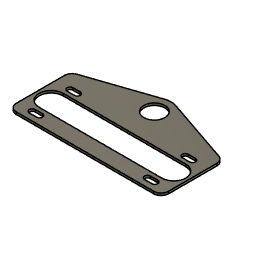
IntakeBack v1 (Autodesk Fusion 360 design; units mm, degrees)
Autodesk Fusion 360 part; units mm, degrees
note: some values were not read from the file. Set by a fixed rule: which sketch regions a step uses.
sketch "Sketch1" plane through (0, 0, 0) normal (0, 1, 0) x (1, 0, 0)
  circle A0 centre (-75, 25) radius 4
  circle A1 centre (-75, -25.8) radius 4
  circle A2 centre (90.1, 25) radius 4
  circle A3 centre (90.1, -25.8) radius 4
  circle A4 centre (-75, -0.4) radius 14.224
  circle A5 centre (90.1, -0.4) radius 14.224
  circle A6 centre (7.55, 56.0402) radius 14.224
  line L0 (-95, -37.4041) -> (-95, 45)
  line L1 (-95, 45) -> (110.1, 45)
  line L2 (110.1, 45) -> (110.1, -45.8)
  circle A7 centre (7.55, 56.0402) radius 22.5
  line L3 (-95, 45) -> (0.3196, 77.3468)
  line L4 (110.1, 45) -> (14.7804, 77.3468)
  line L5 (110.1, -45.8) -> (110.1, -37.4041)
  line L6 (110.1, -37.4041) -> (-95, -37.4041)
  line L7 (90.1, -25.8) -> (86.1, -25.8)
  line L8 (-71, -25.8) -> (-75, -25.8)
  line L9 (-75, 25) -> (-75, 21)
  line L10 (-75, -25.8) -> (-75, -21.8)
  line L11 (-75, 13.824) -> (-75, 25)
  line L12 (-75, 25) -> (-71, 25)
  line L13 (86.1, 25) -> (90.1, 25)
  arc A8 (14.7226, 43.7571) -> (14.1002, 45) centre (-75, -0.4) ccw
  arc A9 (0.9998, 45) -> (0.3774, 43.7571) centre (90.1, -0.4) ccw
  line L14 (90.1, 25) -> (90.1, 21)
  line L15 (90.1, -21.8) -> (90.1, -25.8)
  dimension "d1" = 8
  dimension "d2" = 50.8
  dimension "d3" = 8
  dimension "d4" = 165.1
  dimension "d5" = 50.8
  dimension "d6" = 8
  dimension "d7" = 8
  dimension "d8" = 28.448
  dimension "d9" = 28.448
  dimension "d10" = 200
  dimension "d12" = 28.448
  dimension "d14" = 45
  constraint coincident A0.centre L9.start
  constraint vertical L9
  constraint horizontal L12
  constraint vertical L14
  constraint horizontal L7
  constraint vertical L10
  constraint coincident A2.centre L13.end
  constraint coincident A3.centre L7.start
  constraint concentric A4 A8
  constraint coincident A6.centre A8
  constraint concentric A6 A7
  constraint coincident A7 L3.end
  constraint tangent A7 L3
  constraint coincident A7 L4.end
  constraint tangent A7 L4
  constraint vertical L5
  constraint horizontal L6
  constraint coincident L2 L5.end
  constraint coincident A3 L7.end
  constraint collinear L7 L8
  constraint coincident A1 L8.start
  constraint coincident A4.centre L9
  constraint coincident A4 L11.start
  constraint collinear L10 L11
  constraint coincident A1 L10.end
  constraint coincident A0 L9.end
  constraint coincident A0 L12.end
  constraint collinear L12 L13
  constraint coincident A2 L13.start
  constraint coincident A6 A9.end
  constraint coincident A6 A8.start
  constraint coincident L1 A8.end
  constraint coincident L1 A9.start
  constraint coincident A2 L14.end
  constraint collinear L14 L15
  constraint coincident A5.centre L14
  constraint coincident A3 L15.start
  measures "d1" diameter of A0
  measures "d2" distance of A0.centre A1.centre
  measures "d3" diameter of A1
  measures "d4" distance of A0.centre A2.centre
  measures "d5" distance of A0.centre A1.centre
  measures "d6" diameter of A2
  measures "d7" diameter of A3
  measures "d8" diameter of A4
  measures "d9" diameter of A5
  measures "d10" diameter of A8
  measures "d12" diameter of A6
  measures "d14" diameter of A7
extrude "Extrude1" add sketch "Sketch1" along normal blind 3 contours A6 L1 A7 | A6 L1 A7 | L0 L1 L2 A7 L6 | L1 A7 L3 | L1 A7 L4
sketch "Sketch2" plane through (0, 3, 0) normal (0, 1, 0) x (-1, 0, 0)
  circle A0 centre (-90.1, -25) radius 4
  circle A1 centre (-90.1, 0.4) radius 14.224
  circle A2 centre (75, -25) radius 4
  circle A3 centre (75, 25.8) radius 4
  circle A4 centre (75, 0.4) radius 14.224
  circle A5 centre (-90.1, 25.8) radius 4
  circle A6 centre (-7.55, -56.0402) radius 14.224
  line L0 (-110.1, -45) -> (-14.7804, -77.3468)
  arc A7 (-14.7804, -77.3468) -> (-0.3196, -77.3468) centre (-7.55, -56.0402) ccw
  line L1 (-0.3196, -77.3468) -> (95, -45)
  line L2 (95, -45) -> (95, 37.4041)
  line L3 (95, 37.4041) -> (-110.1, 37.4041)
  line L4 (-110.1, 37.4041) -> (-110.1, -45)
  line L5 (75.0984, -13.8237) -> (-90.1, -13.824)
  line L6 (-90.1, 14.624) -> (75, 14.624)
  constraint coincident A4 L5.start
  constraint coincident A1 L5.end
  constraint tangent A1 L5
  constraint coincident A1 L6.start
  constraint coincident A4 L6.end
  constraint tangent A4 L6
  constraint horizontal L6
extrude "Extrude2" cut sketch "Sketch2" against normal blind 10 contours A1 A4 L5 L6
sketch "Sketch3" plane through (0, 3, 0) normal (0, 1, 0) x (-1, 0, 0)
  line L0 (74.9016, -13.8237) -> (-90.1, -13.824)
  arc A0 (-90.1, 14.624) -> (-90.1, -13.824) centre (-90.1, 0.4) ccw
  line L1 (-90.1, 14.624) -> (75, 14.624)
  arc A1 (74.9016, -13.8237) -> (75, 14.624) centre (75, 0.4) ccw
  circle A2 centre (-90.1, -25) radius 4
  circle A3 centre (75, -25) radius 4
  circle A4 centre (75, 25.8) radius 4
  circle A5 centre (-90.1, 25.8) radius 4
  circle A6 centre (-7.55, -56.0402) radius 14.224
  line L2 (-110.1, -45) -> (-14.7804, -77.3468)
  arc A7 (-14.7804, -77.3468) -> (-0.3196, -77.3468) centre (-7.55, -56.0402) ccw
  line L3 (-0.3196, -77.3468) -> (95, -45)
  line L4 (95, -45) -> (95, 37.4041)
  line L5 (95, 37.4041) -> (-110.1, 37.4041)
  line L6 (-110.1, 37.4041) -> (-110.1, -45)
  arc A8 (-90.1, 16.624) -> (-90.1, -15.824) centre (-90.1, 0.4) ccw
  line L7 (74.8949, -15.8237) -> (-90.1, -15.824)
  arc A9 (74.8949, -15.8237) -> (75, 16.624) centre (75, 0.4) ccw
  line L8 (-90.1, 16.624) -> (75, 16.624)
  dimension "d19" = -2
extrude "Extrude3" cut sketch "Sketch3" against normal blind 10 contours A8 L7 A9 L8
fillet "Fillet1" radius 10 4 edges at (-95, 1.5, 37.4041) (110.1, 1.5, 37.4041) (110.1, 1.5, -45) (-95, 1.5, -45)
sketch "Sketch4" plane through (0, 3, 0) normal (0, 1, 0) x (-1, 0, 0)
  arc A0 (88.2135, -47.303) -> (95, -37.8334) centre (85, -37.8334) ccw
  line L0 (95, -37.8334) -> (95, 27.4041)
  arc A1 (95, 27.4041) -> (85, 37.4041) centre (85, 27.4041) ccw
  line L1 (85, 37.4041) -> (-100.1, 37.4041)
  arc A2 (-100.1, 37.4041) -> (-110.1, 27.4041) centre (-100.1, 27.4041) ccw
  line L2 (-110.1, 27.4041) -> (-110.1, -37.8334)
  arc A3 (-110.1, -37.8334) -> (-103.3135, -47.303) centre (-100.1, -37.8334) ccw
  line L3 (-103.3135, -47.303) -> (-14.7804, -77.3468)
  arc A4 (-14.7804, -77.3468) -> (-0.3196, -77.3468) centre (-7.55, -56.0402) ccw
  line L4 (-0.3196, -77.3468) -> (88.2135, -47.303)
  line L5 (-90.1, 16.624) -> (75, 16.624)
  arc A5 (74.8949, -15.8237) -> (75, 16.624) centre (75, 0.4) ccw
  line L6 (74.8949, -15.8237) -> (-90.1, -15.824)
  arc A6 (-90.1, 16.624) -> (-90.1, -15.824) centre (-90.1, 0.4) ccw
  circle A7 centre (-90.1, -25) radius 4
  circle A8 centre (75, -25) radius 4
  circle A9 centre (75, 25.8) radius 4
  circle A10 centre (-90.1, 25.8) radius 4
  circle A11 centre (-7.55, -56.0402) radius 14.224
  line L7 (75, -25) -> (65, -25)
  circle A12 centre (65, -25) radius 4
  line L8 (75, 25.8) -> (65, 25.8)
  circle A13 centre (65, 25.8) radius 4
  line L9 (-90.1, 25.8) -> (-80.1, 25.8)
  circle A14 centre (-80.1, 25.8) radius 4
  line L10 (-90.1, -25) -> (-80.1, -25)
  circle A15 centre (-80.1, -25) radius 4
  line L11 (75, -29) -> (65, -29)
  line L12 (65, -21) -> (75, -21)
  line L13 (65, 21.8) -> (75, 21.8)
  line L14 (75, 29.8) -> (65, 29.8)
  line L15 (-80.1, 21.8) -> (-90.1, 21.8)
  line L16 (-90.0995, 29.8) -> (-80.1, 29.8)
  line L17 (-90.0995, -21) -> (-80.1, -21)
  line L18 (-80.1, -29) -> (-90.1, -29)
  dimension "d24" = 10
  dimension "d25" = 8
  dimension "d26" = 10
  dimension "d27" = 8
  dimension "d28" = 10
  dimension "d29" = 8
  dimension "d30" = 10
  dimension "d31" = 8
  constraint coincident A8.centre L7.start
  constraint horizontal L7
  constraint coincident L7.end A12.centre
  constraint coincident A9.centre L8.start
  constraint horizontal L8
  constraint coincident L8.end A13.centre
  constraint coincident A10.centre L9.start
  constraint parallel L5 L9
  constraint coincident L9.end A14.centre
  constraint coincident A7.centre L10.start
  constraint horizontal L10
  constraint coincident L10.end A15.centre
  constraint coincident A8 L11.start
  constraint coincident A12 L11.end
  constraint tangent A12 L11
  constraint parallel L7 L11
  constraint coincident A12 L12.start
  constraint coincident A8 L12.end
  constraint tangent A8 L12
  constraint parallel L7 L12
  constraint coincident A13 L13.start
  constraint coincident A9 L13.end
  constraint tangent A9 L13
  constraint parallel L5 L13
  constraint coincident A9 L14.start
  constraint coincident A13 L14.end
  constraint tangent A13 L14
  constraint parallel L8 L14
  constraint coincident A14 L15.start
  constraint coincident A10 L15.end
  constraint tangent A10 L15
  constraint parallel L14 L15
  constraint coincident A10 L16.start
  constraint coincident A14 L16.end
  constraint tangent A14 L16
  constraint parallel L9 L16
  constraint coincident A7 L17.start
  constraint coincident A15 L17.end
  constraint tangent A15 L17
  constraint coincident A15 L18.start
  constraint coincident A7 L18.end
  constraint tangent A7 L18
  constraint parallel L10 L18
  measures "d24" distance of A8.centre L7.end
  measures "d25" diameter of A12
  measures "d26" distance of A9.centre L8.end
  measures "d27" diameter of A13
  measures "d28" distance of A10.centre L9.end
  measures "d29" diameter of A14
  measures "d30" distance of A7.centre L10.end
  measures "d31" diameter of A15
extrude "Extrude4" cut sketch "Sketch4" against normal blind 10 contours A7 L10 A15 L18 | A7 L10 A15 L17 | A15 | A8 L7 A12 L12 | A8 L7 A12 L11 | A12 | A9 L8 A13 L14 | A9 L8 A13 L13 | A13 | A10 L9 A14 L15 | A10 L9 A14 L16 | A14
